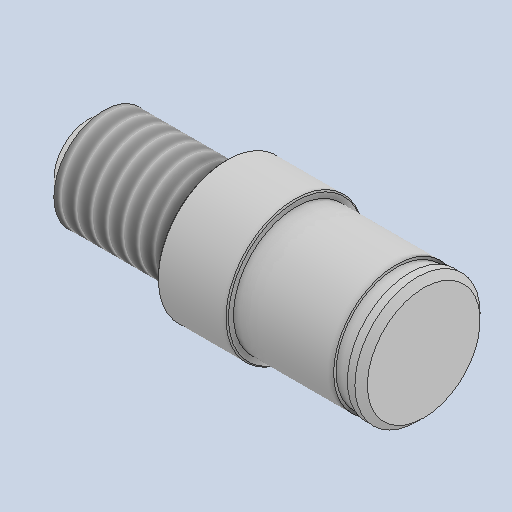
# Autodesk Inventor part: ParallelMech_SupportLink_Proximal_JointShaft
Saved by Autodesk Inventor 2022 (Build 260153000, 153)
## iProperties
Created: 2022-07-30
Part Number: ParallelMech_SupportLink_Proximal_JointShaft
Material: Generisch
Document SubType Name: Modeling
Designer: alexw
Density: 1 g/cm^3
Appearance: Vorgabe
Mass: 1.85771 g
Surface Area: 9.57386 cm^2
Volume: 1.85771 cm^3
Author: alexw
Autodesk Inventor part; units mm, degrees
ref_plane "YZ Plane" through (0, 0, 0) normal (1, 0, 0) x (0, 1, 0)
ref_plane "XZ Plane" through (0, 0, 0) normal (0, 1, 0) x (-1, 0, 0)
ref_plane "XY Plane" through (0, 0, 0) normal (0, 0, 1) x (1, 0, 0)
sketch "Skizze1" plane through (0, 0, 0) normal (0, 0, 1) x (1, 0, 0)
  line L0 (0, 0) -> (0, 5.5)
  line L1 (0, 5.5) -> (5.6, 5.5)
  line L2 (5.6, 5.5) -> (5.6, 5)
  line L3 (5.6, 5) -> (13.6, 5)
  line L4 (13.6, 5) -> (13.6, 4.8)
  line L5 (13.6, 4.8) -> (14.7, 4.8)
  line L6 (14.7, 4.8) -> (14.7, 5)
  line L7 (14.7, 5) -> (15.3, 5)
  line L8 (15.8, 4.5) -> (15.8, 0)
  line L9 (15.8, 0) -> (0, 0)
  line L10 (0, 4) -> (-9.75, 4)
  line L11 (-11, 2.75) -> (-11, 0)
  line L12 (-11, 0) -> (0, 0)
  line L13 (15.3, 5) -> (15.8, 4.5)
  line L14 (-11, 2.75) -> (-9.75, 4)
  line L15 (1.5, 5.5) -> (1.5, 0) construction
  line L16 (13.6, 5) -> (13.6, 0) construction
  line L17 (4.6, 5.5) -> (4.6, 6)
  line L18 (4.6, 6) -> (0, 6)
  line L19 (0, 6) -> (0, 5.5)
  point P0 (15.8, 5)
  point P1 (-11, 4)
  dimension "d0" = 9.6
  dimension "d1" = 0.5
  dimension "d2" = 0.5
  dimension "d3" = 1.1
  dimension "d4" = 10
  dimension "d5" = 0.6
  dimension "d6" = 11
  dimension "d8" = 8
  dimension "d9" = 1.25
  dimension "d10" = 1.25
  dimension "d11" = 11
  dimension "d12" = 4.1
  dimension "d13" = 1.5
  dimension "d14" = 12.1
  dimension "d15" = 0
  dimension "d22" = 1
  dimension "d23" = 12
  constraints: 40 end point, 14 perpendicular, 12 point on line, 2 vertical, 1 collinear
  measures "d0" diameter of L5 L9
  measures "d1" distance of L7.end point (15.8, 5)
  measures "d2" distance of L8.start point (15.8, 5)
  measures "d3" distance between parallel lines of L6 L4
  measures "d4" diameter of L3 L9
  measures "d5" distance from line of L7.end L6
  measures "d6" diameter of L1 L9
  measures "d8" diameter of L10 L12
  measures "d9" distance of L11.start point (-11, 4)
  measures "d10" distance of L10.end point (-11, 4)
  measures "d11" distance between parallel lines of L0 L11
  measures "d12" distance between parallel lines of L2 L15
  measures "d13" distance between parallel lines of L0 L15
  measures "d14" distance between parallel lines of L16 L15
  measures "d15" distance from line of L16 L3.end
  measures "d22" distance between parallel lines of L2 L17
  measures "d23" diameter of L18 L9
revolve "Umdrehung1" add sketch "Skizze1" angle 360 about axis through (15.8, 0, 0) along (-1, 0, 0) contours L12 L11 L14 L10 L0 | L0 L1 L2 L3 L4 L5 L6 L7 L13 L8 L9
thread "Gewinde1" size "M8x1.25" class "6g" standard "ANSI Metric M Profile" full length
chamfer "Fase1" distance 0.1 angle 45 2 edges at (5.6, -5.5, 0) (0, -5.5, 0)
equation "\"d2\" = d1"
equation "\"d10\" = d9"
equation "\"d12\" = Bearing_StepThickness + SupportLink_Proximal_DistStep_Thickness"
equation "\"d14\" = Link_Thickness + SupportLink_Proximal_DistStep_Thickness"
equation "\"SupportLink_Proximal_DistStep_Thickness\" = 2.1"
equation "\"Bearing_StepThickness\" = 2"
equation "\"Link_Thickness\" = 10"
